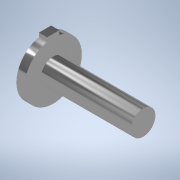
# Autodesk Inventor part: Part35
Saved by Autodesk Inventor 2021 (Build 250183000, 183)
## iProperties
Created: 2020-11-21
Part Number: Part35
Material: Nickel-Copper Alloy 400
Document SubType Name: Modeling
Designer: pedro
Density: 8.83 g/cm^3
Appearance: Chrome - Polished Black
Author: pedro
Autodesk Inventor part; units mm, degrees
ref_plane "YZ Plane" through (0, 0, 0) normal (1, 0, 0) x (0, 1, 0)
ref_plane "XZ Plane" through (0, 0, 0) normal (0, 1, 0) x (-1, 0, 0)
ref_plane "XY Plane" through (0, 0, 0) normal (0, 0, 1) x (1, 0, 0)
sketch "Sketch1" plane through (0, 0, 0) normal (1, 0, 0) x (0, 1, 0)
  circle A0 centre (0, 0) radius 1.5
  circle A1 centre (0, 0) radius 3.5
  circle A2 centre (0, 0) radius 1.5
  line L0 (3.419, -0.7485) -> (3.9058, -0.7485)
  line L1 (3.9058, -0.7485) -> (3.9058, 0.7485)
  line L2 (3.9058, 0.7485) -> (3.419, 0.7485)
  line L3 (3.0942, -0.7485) -> (3.9058, 0.7485) construction
  line L4 (3.9058, -0.7485) -> (3.0942, 0.7485) construction
  point P0 (3.5, 0)
  dimension "d0" = 3
  dimension "d1" = 7
  dimension "d13" = 1.497
  dimension "d16" = 3
  constraints: 10 end point, 3 centre point, 3 point on circle, 2 coincident, 2 midpoint, 1 horizontal, 1 parallel, 1 perpendicular
  measures "d0" diameter of A0
  measures "d1" diameter of A1
  measures "d13" distance of L0.end L1.end
  measures "d16" diameter of A2
extrude "Extrusion1" add sketch "Sketch1" along normal blind 11 contours A0
extrude "Extrusion2" add sketch "Sketch1" against normal blind 1 contours A0 | A1
sketch "Sketch2" plane through (-1, 0, 0) normal (-1, 0, 0) x (0, 0, 1)
  point P0 (0, 0)
extrude "Extrusion3" add sketch "Sketch1" against normal blind 2 contours A0
sketch "Sketch3" plane through (-2, 0, 0) normal (-1, 0, 0) x (0, 0, 1)
  circle A0 centre (0, 0) radius 1
  dimension "d10" = 2
  constraints: 1 centre point, 1 coincident
  measures "d10" diameter of A0
extrude "Extrusion4" cut sketch "Sketch3" against normal blind 1
extrude "Extrusion5" add sketch "Sketch1" against normal blind 1 contours A1 L2 L1 L0
body "Solid1"
